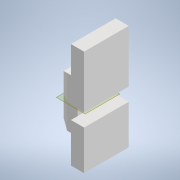
# Autodesk Inventor part: движок
Saved by Autodesk Inventor 2021 (Build 250183000, 183)
## iProperties
Created: 2024-05-11
Part Number: движок
Material: Типовые
Document SubType Name: Modeling
Designer: Мария
Density: 1 g/cm^3
Appearance: По умолчанию
Author: Мария
Autodesk Inventor part; units mm, degrees
ref_plane "YZ Plane" through (0, 0, 0) normal (1, 0, 0) x (0, 1, 0)
ref_plane "XZ Plane" through (0, 0, 0) normal (0, 1, 0) x (-1, 0, 0)
ref_plane "XY Plane" through (0, 0, 0) normal (0, 0, 1) x (1, 0, 0)
sketch "Эскиз1" plane through (0, 0, 0) normal (0, 0, 1) x (1, 0, 0)
  line L0 (-1.6, 0) -> (-1.6, -5.1)
  line L1 (-1.6, -5.1) -> (-4.4, -5.1)
  line L2 (-4.4, -5.1) -> (-4.4, -12.7)
  line L3 (-4.4, -12.7) -> (-1.6, -12.7)
  line L4 (-1.6, -12.7) -> (-1.6, -16)
  line L5 (-1.6, -16) -> (0, -16)
  line L6 (0, -16) -> (0, -10)
  line L7 (0, -10) -> (-1.6, -10)
  line L8 (-1.6, -10) -> (-1.6, -8)
  line L9 (-1.6, -8) -> (0, -8)
  line L10 (-1.6, 0) -> (0, 0)
  line L11 (0, 0) -> (0, -8)
  line L12 (-4.4, -6.4) -> (0, -6.4) construction
  dimension "d1" = 1.6
  dimension "d5" = 2
  dimension "d6" = 10
  dimension "d7" = 8
  dimension "d32" = 2.8
  dimension "d33" = 7.6
  dimension "d34" = 1.6
  dimension "d35" = 2.9
  constraints: 26 end point, 7 perpendicular, 3 vertical alignment, 2 point on line, 2 vertical, 1 coincident, 1 horizontal
  measures "d1" distance between parallel lines of L6 L4
  measures "d5" distance between parallel lines of L7 L9
  measures "d6" distance between parallel lines of L10 L7
  measures "d7" distance between parallel lines of L5 L9
  measures "d32" distance between parallel lines of L0 L2
  measures "d33" distance between parallel lines of L1 L3
  measures "d34" distance between parallel lines of L12 L9
  measures "d35" distance between parallel lines of L1 L9
extrude "Выдавливание1" add sketch "Эскиз1" along normal blind 4.8
ref_plane "РабПлоскость1" through (-4.4, -8.9, 0) normal (0, -1, 0) x (1, 0, 0)
sketch "Эскиз2" plane through (-1.6, -5.1, 0) normal (-1, 0, 0) x (0, 0, 1)
  line L0 (0, -7.6) -> (0, -10.9) projected
  line L1 (0, 5.1) -> (0, 0) projected
  line L2 (4.8, -7.6) -> (4.8, -10.9) projected
  line L3 (0, -7.6) -> (4.8, -7.6) projected
  line L4 (0, -10.9) -> (4.8, -10.9) projected
  line L5 (0, 0) -> (4.8, 0) projected
  line L6 (0, 5.1) -> (4.8, 5.1) projected
  line L7 (4.8, 5.1) -> (4.8, 0) projected
  line L8 (-1, -10.9) -> (5.8, -10.9)
  line L9 (5.8, -10.9) -> (5.8, -4.9)
  line L10 (5.8, -4.9) -> (-1, -4.9)
  line L11 (-1, -4.9) -> (-1, -10.9)
  line L12 (-1, -2.9) -> (5.8, -2.9)
  line L13 (5.8, -2.9) -> (5.8, 5.1)
  line L14 (5.8, 5.1) -> (-1, 5.1)
  line L15 (-1, 5.1) -> (-1, -2.9)
  line L16 (0, -2.9) -> (4.8, -2.9) projected
  line L17 (0, -4.9) -> (4.8, -4.9) projected
  point P0 (0, 5.1)
  point P1 (4.8, 5.1)
  dimension "d10" = 1
  dimension "d11" = 1
  constraints: 16 end point, 4 horizontal alignment, 4 parallel, 2 horizontal, 2 perpendicular, 2 point on line
  measures "d10" distance between parallel lines of L11 L0
  measures "d11" distance between parallel lines of L2 L9
extrude "Выдавливание2" add sketch "Эскиз2" against normal up to surface (1.6 mm away) contours L0 L8 L11 L10 L9 L2 L3 | L1 L5 L7 L14 L13 L12 L15
chamfer "Фаска6" distance 0.7 angle 60 4 edges at (-4.4, -8.9, 4.8) (-4.4, -12.7, 2.4) (-4.4, -5.1, 2.4) (-4.4, -8.9, 0) measured on face at (-4.4, -12.2, 2.4) measured on face at (-4.4, -8.9, 4.3) measured on face at (-4.4, -8.9, 0.5) measured on face at (-4.4, -5.6, 2.4)
